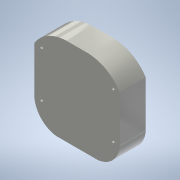
# Autodesk Inventor part: pcb
Saved by Autodesk Inventor 2021 (Build 250183000, 183)
## iProperties
Created: 2015-03-17
Part Number: pcb
Material: Générique
Document SubType Name: Modeling
Designer: sd
Density: 1 g/cm^3
Appearance: Lisse - Ivoire
Author: sd
Autodesk Inventor part; units mm, degrees
ref_plane "YZ Plane" through (0, 0, 0) normal (1, 0, 0) x (0, 1, 0)
ref_plane "XZ Plane" through (0, 0, 0) normal (0, 1, 0) x (-1, 0, 0)
ref_plane "XY Plane" through (0, 0, 0) normal (0, 0, 1) x (1, 0, 0)
sketch "Esquisse1" plane through (0, 0, 0) normal (0, 1, 0) x (-1, 0, 0)
  line L0 (-43, -44) -> (43, -44)
  line L1 (43, -44) -> (43, 44)
  line L2 (43, 44) -> (-43, 44)
  line L3 (-43, 44) -> (-43, -44)
  point P0 (0, 0)
  dimension "d0" = 86
  dimension "d1" = 88
  dimension "d2" = 43
  dimension "d3" = 44
  constraints: 8 end point, 2 parallel, 1 horizontal, 1 perpendicular
  measures "d0" distance of L1.end L2.end
  measures "d1" distance of L2.end L0.start
  measures "d2" horizontal distance of point (0, 0) L2.end
  measures "d3" vertical distance of point (0, 0) L2.end
extrude "Carre de base" add sketch "Esquisse1" along normal blind 26
sketch "Esquisse2" plane through (0, 26, 0) normal (0, 1, 0) x (1, 0, 0)
  line L0 (43, 44) -> (-43, 44) projected
  line L1 (-43, 44) -> (-43, -44) projected
  line L2 (-43, -44) -> (43, -44) projected
  line L3 (43, -44) -> (43, 44) projected
  line L4 (-43, -21) -> (-43, -26)
  line L5 (43, -21) -> (43, -26)
  line L6 (-43, 14) -> (-43, 19)
  line L7 (43, 14) -> (43, 19)
  line L8 (10, -44) -> (-10, -44)
  line L9 (21, 44) -> (-21, 44)
  arc A0 (10, -44) -> (43, -26) centre (10, -4.75) ccw
  arc A1 (-43, -26) -> (-10, -44) centre (-10, -4.75) ccw
  arc A2 (43, 19) -> (21, 44) centre (17.7955, 19) ccw
  arc A3 (-21, 44) -> (-43, 19) centre (-17.7955, 19) ccw
  line L10 (-43, -21) -> (-43, 14)
  line L11 (43, -21) -> (43, 14)
  point P0 (0, 0)
  dimension "d13" = 5
  dimension "d14" = 5
  dimension "d15" = 5
  dimension "d16" = 5
  dimension "d21" = 20
  dimension "d22" = 10
  dimension "d23" = 42
  dimension "d24" = 21
  dimension "d25" = 39.25
  dimension "d26" = 39.25
  dimension "d27" = 25.2046
  dimension "d28" = 25.2046
  dimension "d74" = 35
  dimension "d75" = 35
  dimension "d76" = 18
  dimension "d77" = 18
  constraints: 16 end point, 12 point on line, 8 point on circle, 4 centre point, 2 collinear, 2 tangent
  measures "d13" distance of L5.start L5.end
  measures "d14" distance of L4.start L4.end
  measures "d15" distance of L7.start L7.end
  measures "d16" distance of L6.start L6.end
  measures "d21" distance of L8.start L8.end
  measures "d22" horizontal distance of point (0, 0) L8.start
  measures "d23" distance of L9.start L9.end
  measures "d24" horizontal distance of point (0, 0) L9.start
  measures "d25" radius of A0
  measures "d26" radius of A1
  measures "d27" radius of A2
  measures "d28" radius of A3
  measures "d74" distance of L7.start L5.start
  measures "d75" distance of L6.start L4.start
  measures "d76" vertical distance of L8.end L4.end
  measures "d77" distance of L2.end L5.end
sketch "Esquisse6" plane through (0, 26, 0) normal (0, 1, 0) x (1, 0, 0)
  circle A0 centre (36, -26) radius 1.6
  circle A1 centre (-36, -26) radius 1.6
  circle A2 centre (-36, 20) radius 1.6
  circle A3 centre (36, 20) radius 1.6
  point P0 (0, 0)
  dimension "d59" = 3.2
  dimension "d60" = 3.2
  dimension "d61" = 3.2
  dimension "d62" = 3.2
  dimension "d63" = 36
  dimension "d64" = 36
  dimension "d65" = 36
  dimension "d66" = 36
  dimension "d67" = 26
  dimension "d68" = 26
  dimension "d69" = 20
  dimension "d70" = 20
  constraints: 4 centre point
  measures "d59" diameter of A3
  measures "d60" diameter of A2
  measures "d61" diameter of A0
  measures "d62" diameter of A1
  measures "d63" horizontal distance of point (0, 0) A0.centre
  measures "d64" horizontal distance of point (0, 0) A1.centre
  measures "d65" horizontal distance of point (0, 0) A3.centre
  measures "d66" horizontal distance of point (0, 0) A2.centre
  measures "d67" vertical distance of point (0, 0) A0.centre
  measures "d68" vertical distance of point (0, 0) A1.centre
  measures "d69" vertical distance of point (0, 0) A3.centre
  measures "d70" vertical distance of point (0, 0) A2.centre
extrude "Extrusion7" cut sketch "Esquisse6" against normal through all
extrude "Extrusion8" cut sketch "Esquisse2" against normal through all contours L3 A2 L0 | A3 L1 L0 | L3 L2 A0 | A1 L2 L1
equation "\"d2\" = 0.5 * d0"
equation "\"d3\" = 0.5 * d1"
equation "\"d13\" = d14"
equation "\"d15\" = d16"
equation "\"d22\" = 0.5 * d21"
equation "\"d24\" = 0.5 * d23"
equation "\"d26\" = d25"
equation "\"d28\" = d27"
equation "\"d60\" = d59"
equation "\"d61\" = d59"
equation "\"d62\" = d59"
equation "\"d64\" = d63"
equation "\"d65\" = d63"
equation "\"d66\" = d63"
equation "\"d68\" = d67"
